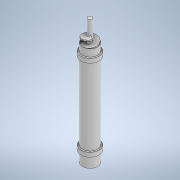
# Autodesk Inventor part: Arkimedes skruv
Saved by Autodesk Inventor 2021 (Build 250183000, 183)
## iProperties
Created: 2024-12-11
Part Number: Arkimedes skruv
Material: Generic
Document SubType Name: Modeling
Designer: 24lucsil
Density: 1 g/cm^3
Appearance: Default
Author: 24lucsil
Autodesk Inventor part; units mm, degrees
ref_plane "YZ Plane" through (0, 0, 0) normal (1, 0, 0) x (0, 1, 0)
ref_plane "XZ Plane" through (0, 0, 0) normal (0, 1, 0) x (-1, 0, 0)
ref_plane "XY Plane" through (0, 0, 0) normal (0, 0, 1) x (1, 0, 0)
sketch "Sketch1" plane through (0, 0, 0) normal (0, 1, 0) x (-1, 0, 0)
  circle A0 centre (0, 0) radius 65.1659
  circle A1 centre (0, 0) radius 3
  dimension "d0" = 6
  constraints: 2 centre point, 2 coincident
  measures "d0" diameter of A1
extrude "Extrusion1" add sketch "Sketch1" along normal blind 175 contours A1
sketch "Sketch2" plane through (0, 0, 0) normal (0, 0, 1) x (1, 0, 0)
  line L0 (3, 0) -> (-3, 0) projected
  line L1 (-3, 0) -> (-10, 0)
  line L2 (-10, 0) -> (-10, 1.5)
  line L3 (-10, 1.5) -> (-3, 1.5)
  line L4 (-3, 1.5) -> (-3, 0)
  point P0 (0, 0)
  dimension "d3" = 7
  dimension "d4" = 1.5
  constraints: 8 end point, 2 parallel, 1 horizontal, 1 perpendicular
  measures "d3" distance of L0.end L1.end
  measures "d4" distance of L1.end L2.end
coil "Coil1" sketch "Sketch2" operation add axis through (0, -10, 0) along (0, 1, 0) pitch 10 turns 15.415 hand right
sketch "Sketch3" plane through (0, 0, 0) normal (0, -1, 0) x (1, 0, 0)
  circle A0 centre (0, 0) radius 10
  circle A1 centre (0, 0) radius 10.75
  dimension "d13" = 20
  dimension "d14" = 21.5
  constraints: 2 centre point, 2 coincident
  measures "d13" diameter of A0
  measures "d14" diameter of A1
extrude "Extrusion2" add sketch "Sketch3" against normal blind 145
sketch "Sketch4" plane through (0, 0, 0) normal (0, 0, 1) x (1, 0, 0)
  line L0 (-10.75, 0) -> (10.75, 0) projected
  line L1 (-10.75, 0) -> (-10.75, 15)
  line L2 (-10.75, 0) -> (-10.75, 145) projected
  line L3 (-10.75, 15) -> (-12.75, 15)
  line L4 (-12.75, 15) -> (-12.75, 21)
  line L5 (-12.75, 21) -> (-10.75, 21)
  line L6 (-10.75, 21) -> (-10.75, 15)
  line L7 (0, -35) -> (0, 210) projected
  point P0 (0, 0)
  dimension "d17" = 15
  dimension "d18" = 2
  dimension "d19" = 6
  constraints: 10 end point, 2 parallel, 1 horizontal, 1 perpendicular, 1 point on line
  measures "d17" distance of L0.start L1.end
  measures "d18" distance of L4.end L5.end
  measures "d19" distance of L3.end L4.end
revolve "Revolution1" add sketch "Sketch4" angle 360 about axis through (0, -10, 0) along (0, 1, 0)
sketch "Sketch5" plane through (0, 0, 0) normal (0, 0, 1) x (1, 0, 0)
  line L0 (10.75, 145) -> (-10.75, 145) projected
  line L1 (-10.75, 145) -> (-10.75, 135)
  line L2 (-10.75, 21) -> (-10.75, 145) projected
  line L3 (-10.75, 135) -> (-12.75, 135)
  line L4 (-12.75, 135) -> (-12.75, 129)
  line L5 (-12.75, 129) -> (-10.75, 129)
  line L6 (-10.75, 129) -> (-10.75, 135)
  line L7 (0, -35) -> (0, 210) projected
  point P0 (0, 0)
  dimension "d21" = 10
  dimension "d22" = 6
  dimension "d23" = 2
  constraints: 10 end point, 2 parallel, 1 horizontal, 1 perpendicular, 1 point on line
  measures "d21" distance of L0.end L1.end
  measures "d22" distance of L3.end L4.end
  measures "d23" distance of L4.end L5.end
revolve "Revolution2" add sketch "Sketch5" angle 360 about axis through (0, -10, 0) along (0, 1, 0)
body "Solid1"
